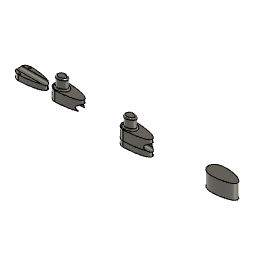
line holder parts (Autodesk Fusion 360 design; units mm, degrees)
Autodesk Fusion 360 part; units mm, degrees
note: some values were not read from the file. Set by a fixed rule: which sketch regions a step uses; which face or edge a step refers to.
sketch "Sketch2" plane through (0, 0, 0) normal (0, 0, 1) x (1, 0, 0)
  line L0 (10, 10) -> (10.0021, 10)
  line L1 (44.9955, 0.0036) -> (44.9955, 0.0036)
  line L2 (44.9955, 0.0036) -> (44.9955, -0.0645)
  line L3 (10.0013, -10) -> (10, -10)
  arc A0 (10, 10) -> (10, -10) centre (10, 0) ccw
  spline S0 degree 5 poles (10, 10) (10.0476, 10.0003) (10.826, 9.9636) (14.0429, 9.7956) (21.7538, 9.2439) (33.4763, 7.503) (43.0429, 4.4199) (46.8335, 0.0034) (43.1596, -4.4135) (33.7029, -7.4977) (22.0372, -9.2403) (14.2896, -9.7934) (10.9779, -9.9626) (10.1037, -10) (10, -10) knots 0 0 0 0 0 0 0.1 0.2 0.3 0.4 0.5 0.6 0.7 0.8 0.9 1 1 1 1 1 1
  line L4 (9.8556, 9.999) -> (10.1444, 10.001)
  line L5 (10.315, -10) -> (9.685, -10)
  line L6 (44.9689, 1.9602) -> (45.0221, -1.953)
  dimension "d6" = 20
  constraint perpendicular L0 L1
  constraint perpendicular L0 L2
  constraint perpendicular L2 L3
  constraint midpoint L0.start L4
  constraint midpoint L3.end L5
  constraint coincident S0 L0.end
  constraint coincident S0 L1.start
  constraint coincident S0 L3.start
  constraint coincident S0 L2.end
  constraint midpoint L1.start L6
  measures "d6" diameter of A0
extrude "Extrude1" add sketch "Sketch2" along normal blind 15 makes body 1
sketch "Sketch3" plane through (0, 0, 15) normal (0, 0, 1) x (-1, 0, 0)
  arc A0 (-10, -10) -> (-10, 10) centre (-10, 0) ccw
  line L0 (-10, 10) -> (-10.0013, 10)
  spline S0 degree 5 poles (-10.0013, 10) (-10.1082, 9.9998) (-10.9865, 9.9622) (-14.2996, 9.7927) (-22.0433, 9.2394) (-33.6661, 7.5031) (-41.2087, 5.0497) (-44.2915, 2.6186) (-44.9856, 0.912) (-44.9955, 0.0645) knots -0.99974 -0.99974 -0.99974 -0.99974 -0.99974 -0.99974 -0.9 -0.8 -0.7 -0.6 -0.501575 -0.501575 -0.501575 -0.501575 -0.501575 -0.501575
  line L1 (-44.9955, 0.0645) -> (-44.9955, -0.0036)
  spline S1 degree 5 poles (-44.9955, -0.0036) (-44.9838, -0.8647) (-44.2701, -2.5868) (-41.1293, -5.0366) (-33.4762, -7.503) (-21.7722, -9.2412) (-14.0733, -9.7934) (-10.8514, -9.9623) (-10.06, -9.9998) (-10.0021, -10) knots -0.499993 -0.499993 -0.499993 -0.499993 -0.499993 -0.499993 -0.4 -0.3 -0.2 -0.1 -0.000788 -0.000788 -0.000788 -0.000788 -0.000788 -0.000788
  line L2 (-10.0021, -10) -> (-10, -10)
  spline S2 degree 5 poles (-3.5, 0) (-3.503, -0.4404) (-3.5965, -1.3221) (-3.9989, -2.6214) (-5.001, -4.2028) (-6.7223, -5.6915) (-8.6437, -6.5249) (-10.5895, -6.6249) (-12.8813, -6.089) (-15.4481, -5.0387) (-17.8747, -3.5902) (-19.6465, -1.8683) (-20.3024, -0.0013) (-19.6285, 1.8751) (-17.8371, 3.6173) (-15.3884, 5.0811) (-12.7997, 6.1281) (-10.4886, 6.6359) (-8.5437, 6.4995) (-6.639, 5.6556) (-4.9418, 4.1781) (-3.9627, 2.6124) (-3.5783, 1.3205) (-3.497, 0.4404) (-3.5, 0) knots 0 0 0 0 0 0 0.05 0.1 0.15 0.2 0.25 0.3 0.35 0.4 0.45 0.5 0.55 0.6 0.65 0.7 0.75 0.8 0.85 0.9 0.95 1 1 1 1 1 1
  line L3 (-11.8068, 6.5289) -> (-7.9909, 6.4695)
  line L4 (-8.1367, -6.5144) -> (-11.9622, -6.4853)
  point P0 (-10.0495, -6.4998)
  point P1 (-19.9735, 0)
  point P2 (-9.8988, 6.4992)
  constraint midpoint P2 L3
  constraint midpoint P0 L4
extrude "Extrude2" add sketch "Sketch3" along normal blind 15 contours S2 bodies 1
fillet "Fillet1" radius 2 1 faces at (9.5802, 1.5094, 30) on bodies 1
fillet "Fillet2" radius 2 1 edges at (19.9735, -0.001, 15) on bodies 1
extrude "Extrude3" add 1 faces at (17.7989, 3.0952, 0) along direction (0, 0, -1) blind 8 separate body on bodies 1 makes body 2
hole "Hole1" at (0, 0, 3.9635) direction (1, 0, 0) diameter 12 depth 50 tip angle 118 bodies 1 2
hole "Hole2" at (10.075, -7.9165, -8) direction (0, 0, 1) diameter 2 depth 20 tip angle 118 bodies 1 2
hole "Hole3" at (9.8923, 8.0383, -8) direction (0, 0, 1) diameter 2 depth 20 tip angle 118 bodies 1 2
hole "Hole4" at (10.075, -7.9165, -8) direction (0, 0, 1) diameter 3 depth 8 tip angle 180 bodies 2
hole "Hole5" at (9.8923, 8.0383, -8) direction (0, 0, 1) diameter 3 depth 8 tip angle 180 bodies 2
copy_body "CopyPasteBodies1" bodies 2 makes body 3
move_body "Move1" bodies 3 to x (1, 0, 0) y (0, 1, 0) z (0, 0, 1) at (-159.6516, 0, 8.3782)
move_body "Move2" bodies 3 to x (1, 0, 0) y (0, 1, 0) z (0, 0, 1) at (-0.3284, 0, -0.3284)
copy_body "CopyPasteBodies2" bodies 1 makes body 4
move_body "Move3" bodies 4 to x (1, 0, 0) y (0, 1, 0) z (0, 0, 1) at (-103.8718, 0, 0.3058)
copy_body "Body->Comp1" bodies 3 removing the originals makes body 5 in component "Component"
copy_body "Body->Comp2" bodies 4 removing the originals makes body 6 in component "Component'"
move_body "Move1'" bodies 6 to x (1, 0, 0) y (0, 1, 0) z (0, 0, 1) at (-0.1501, 0, -0.2502) in component "Component'"
sketch "Sketch4" plane through (0, 0, -8) normal (0, 0, -1) x (1, 0, 0)
  circle A0 centre (9.8923, -8.0383) radius 1.5
  circle A1 centre (10.075, 7.9165) radius 1.5
  arc A2 (10, 10) -> (10, -10) centre (10, 0) ccw
  line L0 (10, -10) -> (10.0021, -10)
  spline S0 degree 5 poles (10.0021, -10) (10.06, -9.9998) (10.8514, -9.9623) (14.0733, -9.7934) (21.7722, -9.2412) (33.4762, -7.503) (41.1293, -5.0366) (44.2701, -2.5868) (44.9838, -0.8647) (44.9955, -0.0036) knots 0.000788 0.000788 0.000788 0.000788 0.000788 0.000788 0.1 0.2 0.3 0.4 0.499993 0.499993 0.499993 0.499993 0.499993 0.499993
  line L1 (44.9955, -0.0036) -> (44.9955, 0.0645)
  spline S1 degree 5 poles (44.9955, 0.0645) (44.9856, 0.912) (44.2915, 2.6186) (41.2087, 5.0497) (33.6661, 7.5031) (22.0433, 9.2394) (14.2996, 9.7927) (10.9865, 9.9622) (10.1082, 9.9998) (10.0013, 10) knots 0.501575 0.501575 0.501575 0.501575 0.501575 0.501575 0.6 0.7 0.8 0.9 0.99974 0.99974 0.99974 0.99974 0.99974 0.99974
  line L2 (10.0013, 10) -> (10, 10)
  spline S2 degree 5 poles (70, 0) (70, 0.9037) (70.0749, 2.711) (70.4117, 5.3178) (71.5102, 8.1683) (74.7337, 10.0634) (80.3994, 10.1088) (87.8749, 9.7182) (95.9779, 9.6448) (103.7062, 9.3457) (110.0661, 7.9729) (114.2614, 4.8996) (115.7314, 0) (114.2614, -4.8996) (110.0661, -7.9729) (103.7062, -9.3457) (95.9779, -9.6448) (87.8749, -9.7182) (80.3994, -10.1088) (74.7337, -10.0634) (71.5102, -8.1683) (70.4117, -5.3178) (70.0749, -2.711) (70, -0.9037) (70, 0) knots 0 0 0 0 0 0 0.05 0.1 0.15 0.2 0.25 0.3 0.35 0.4 0.45 0.5 0.55 0.6 0.65 0.7 0.75 0.8 0.85 0.9 0.95 1 1 1 1 1 1
  line L3 (74, 10) -> (86, 10)
  line L4 (86, -10) -> (74, -10)
  line L5 (115, 3) -> (115, -3)
  spline S3 degree 5 poles (130.0022, 0.2082) (130.0429, 0.7638) (130.2129, 1.8742) (130.7273, 3.5169) (131.9089, 5.5788) (134.1589, 7.7494) (137.1499, 9.3623) (140.8484, 10.3261) (145.2927, 10.6559) (150.3414, 10.4239) (155.684, 9.7249) (160.9343, 8.6724) (165.6876, 7.3822) (169.5933, 5.9612) (172.4201, 4.4946) (174.1293, 3.0326) (174.9339, 1.579) (175.1121, 0.112) (174.8239, -1.3963) (173.947, -2.9607) (172.2482, -4.5733) (169.5333, -6.1942) (165.8077, -7.7407) (161.2319, -9.1024) (156.0769, -10.1559) (150.6805, -10.7798) (145.4047, -10.8691) (140.5913, -10.3508) (136.5216, -9.1983) (133.3656, -7.4494) (131.1954, -5.1996) (130.2507, -3.1108) (129.9685, -1.4597) (129.9614, -0.3475) (130.0022, 0.2082) knots 0 0 0 0 0 0 0.033333 0.066667 0.1 0.133333 0.166667 0.2 0.233333 0.266667 0.3 0.333333 0.366667 0.4 0.433333 0.466667 0.5 0.533333 0.566667 0.6 0.633333 0.666667 0.7 0.733333 0.766667 0.8 0.833333 0.866667 0.9 0.933333 0.966667 1 1 1 1 1 1
  line L6 (135.2103, 8.9989) -> (145, 11)
  point P0 (80, 10)
  point P1 (115, 0)
  point P2 (80, -10)
  point P3 (140.1051, 9.9994)
  point P4 (172.0175, 4.5749)
  point P5 (174.9957, 0.2082)
  point P6 (171.964, -4.5981)
  point P7 (139.8419, -9.9987)
  dimension "d31" = 44.9955
  dimension "d32" = 20
  dimension "d33" = 10
  constraint midpoint P0 L3
  constraint midpoint P2 L4
  constraint midpoint P1 L5
  constraint midpoint P3 L6
  measures "d31" distance of origin S0.end
  measures "d32" vertical distance of L0.end A2.start
  measures "d33" distance of origin A2.centre
extrude "Extrude4" add sketch "Sketch4" along normal blind 22 separate body contours S3 makes body 7
move_face "MoveFace1" to x (1, 0, 0) y (0, 1, 0) z (0, 0, 1) at (0, 0, 300) 1 faces at (138.5291, -9.6079, -19) on bodies 7
move_face "MoveFace2" to x (1, 0, 0) y (0, 1, 0) z (0, 0, 1) at (0, 0, 30) 1 faces at (138.5291, -9.6079, -19) on bodies 7
move_body "Move4" bodies 7 to x (1, 0, 0) y (0, 1, 0) z (0, 0, 1) at (0, 0, 30.2684)
sketch "Sketch5" plane through (0, 0, 0) normal (0, 0, 1) x (1, 0, 0)
component "Component" placed x (1, 0, 0) y (0, 1, 0) z (0, 0, 1) at (0, 0, 0)
component "Component'" placed x (1, 0, 0) y (0, 1, 0) z (0, 0, 1) at (0, 0, 0)
